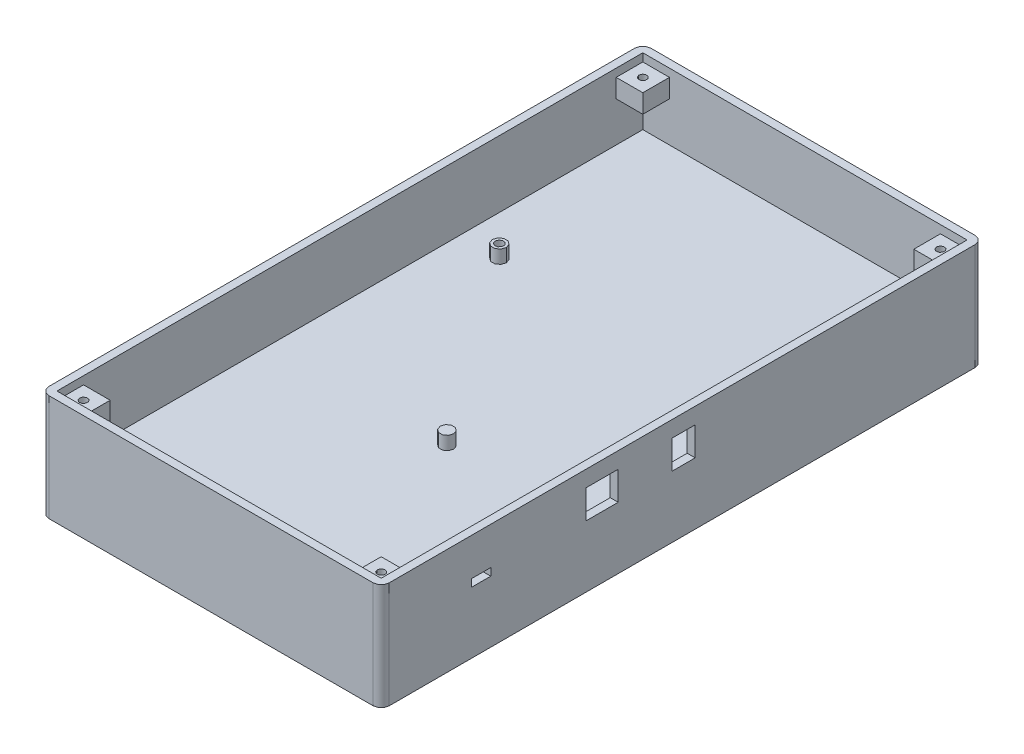
# Autodesk Inventor part: Base
Saved by Autodesk Inventor 2023 (Build 270158000, 158)
## iProperties
Created: 2023-01-13
Part Number: Base
Material: Generic
Document SubType Name: Modeling
Designer: Ahmed Nazir
Density: 1 g/cm^3
Appearance: Default
Author: Ahmed Nazir
Autodesk Inventor part; units mm, degrees
ref_plane "YZ Plane" through (0, 0, 0) normal (1, 0, 0) x (0, 1, 0)
ref_plane "XZ Plane" through (0, 0, 0) normal (0, 1, 0) x (-1, 0, 0)
ref_plane "XY Plane" through (0, 0, 0) normal (0, 0, 1) x (1, 0, 0)
sketch "Sketch1" plane through (0, 0, 0) normal (0, 1, 0) x (-1, 0, 0)
  line L0 (0, 0) -> (121.76, 0)
  line L1 (121.76, 0) -> (121.76, -220)
  line L2 (121.76, -220) -> (0, -220)
  line L3 (0, -220) -> (0, 0)
  line L4 (124.76, -223) -> (124.76, 3)
  line L5 (124.76, 3) -> (-3, 3)
  line L6 (-3, 3) -> (-3, -223)
  line L7 (-3, -223) -> (124.76, -223)
  circle A0 centre (5.08, -10.08) radius 1.6
  circle A1 centre (5.08, -10.08) radius 2.6
  circle A2 centre (55.88, -80.565) radius 2.5
  circle A3 centre (5.08, -151.05) radius 1.6
  circle A4 centre (5.08, -151.05) radius 2.6
  circle A5 centre (106.68, -10.08) radius 1.6
  circle A6 centre (106.68, -10.08) radius 2.6
  circle A7 centre (106.68, -151.05) radius 1.6
  circle A8 centre (106.68, -151.05) radius 2.6
  dimension "d0" = 121.76
  dimension "d1" = 220
  dimension "d2" = 3
  dimension "d22" = 3.2
  dimension "d23" = 1
  dimension "d24" = 5.08
  dimension "d25" = 10.08
  dimension "d26" = 5
  dimension "d35" = 3.2
  dimension "d36" = 1
  dimension "d37" = 140.97
  dimension "d38" = 0
  dimension "d39" = 3.2
  dimension "d40" = 1
  dimension "d41" = 101.6
  dimension "d42" = 0
  dimension "d43" = 3.2
  dimension "d44" = 1
  dimension "d45" = 0
  dimension "d46" = 0
  dimension "d47" = 50.8
  dimension "d48" = 70.485
  constraints: 16 end point, 9 centre point, 4 parallel, 2 perpendicular, 1 horizontal, 3 other
  measures "d0" distance of L1.end L2.end
  measures "d1" distance of L0.end L1.end
  measures "d2" distance between parallel lines of L1 L4
  measures "d22" diameter of A0
  measures "d23" radial gap between concentric circles of A0 A1
  measures "d24" distance from line of L3 A0.centre
  measures "d25" distance from line of A0.centre L0
  measures "d26" diameter of A2
  measures "d35" diameter of A3
  measures "d36" radial gap between concentric circles of A3 A4
  measures "d37" distance of A3.centre A0.centre
  measures "d38" horizontal distance of A3.centre A0.centre
  measures "d39" diameter of A5
  measures "d40" radial gap between concentric circles of A5 A6
  measures "d41" distance of A0.centre A5.centre
  measures "d42" vertical distance of A5.centre A0.centre
  measures "d43" diameter of A7
  measures "d44" radial gap between concentric circles of A7 A8
  measures "d45" vertical distance of A3.centre A7.centre
  measures "d46" horizontal distance of A5.centre A7.centre
  measures "d47" horizontal distance of A2.centre A0.centre
  measures "d48" vertical distance of A2.centre A5.centre
extrude "Extrusion1" add sketch "Sketch1" along normal blind 15 contours L0 L1 L2 L3 | A0 | A1 | A2 | A3 | A4 | A5 | A6 | A7 | A8
extrude "Extrusion2" add sketch "Sketch1" along normal blind 40 contours L7 L6 L5 L4
fillet "Fillet1" radius 3 4 edges at (3, 20, -223) (-124.76, 20, -223) (-124.76, 20, 3) (3, 20, 3)
sketch "Sketch2" plane through (3, 0, 0) normal (1, 0, 0) x (0, 0, -1)
  line L0 (220, 15) -> (0, 15) construction
  line L1 (0, 15) -> (220, 15)
  line L2 (73.9, 33.95) -> (86, 33.95)
  line L3 (86, 33.95) -> (86, 23.2)
  line L4 (86, 23.2) -> (73.9, 23.2)
  line L5 (73.9, 23.2) -> (73.9, 33.95)
  line L6 (106.15, 33.95) -> (114.9, 33.95)
  line L7 (114.9, 33.95) -> (114.9, 23.2)
  line L8 (114.9, 23.2) -> (106.15, 23.2)
  line L9 (106.15, 23.2) -> (106.15, 33.95)
  line L10 (0, 0) -> (0, 40) projected
  line L11 (30.85, 25.9) -> (38.15, 25.9)
  line L12 (38.15, 25.9) -> (38.15, 23.1)
  line L13 (38.15, 23.1) -> (30.85, 23.1)
  line L14 (30.85, 23.1) -> (30.85, 25.9)
  line L15 (110, 15) -> (110, 0) construction
  line L16 (220, 0) -> (0, 0) projected
  line L17 (48.413, 0) -> (43.7499, 10)
  line L18 (43.7499, 10) -> (66.2501, 10)
  line L19 (66.2501, 10) -> (61.587, 0)
  line L20 (48.413, 0) -> (61.587, 0)
  line L21 (55, 0) -> (55, 15) construction
  line L22 (171.587, 0) -> (176.2501, 10)
  line L23 (176.2501, 10) -> (153.7499, 10)
  line L24 (153.7499, 10) -> (158.413, 0)
  line L25 (171.587, 0) -> (158.413, 0)
  point P0 (110, 7.5)
  point P1 (55, 0)
  point P2 (158.413, 0)
  dimension "d9" = 12.1
  dimension "d10" = 10.75
  dimension "d11" = 8.2
  dimension "d12" = 8.75
  dimension "d13" = 10.75
  dimension "d14" = 8.2
  dimension "d15" = 20.15
  dimension "d19" = 7.3
  dimension "d20" = 2.8
  dimension "d21" = 8.1
  dimension "d49" = 35.75
  dimension "d50" = 30.85
  dimension "d72" = 13.174
  dimension "d73" = 65
  dimension "d74" = 65
  dimension "d75" = 10
  dimension "d76" = 55
  constraints: 46 end point, 7 equal length, 5 horizontal, 5 point on line, 4 midpoint, 4 perpendicular, 4 symmetric about line
  measures "d9" distance of L3.end L4.end
  measures "d10" distance of L2.end L3.end
  measures "d11" distance between parallel lines of L0 L4
  measures "d12" distance of L7.end L8.end
  measures "d13" distance of L6.end L7.end
  measures "d14" distance between parallel lines of L0 L8
  measures "d15" distance between parallel lines of L9 L3
  measures "d19" distance of L12.end L13.end
  measures "d20" distance of L11.end L12.end
  measures "d21" distance between parallel lines of L0 L13
  measures "d49" distance between parallel lines of L5 L12
  measures "d50" distance between parallel lines of L10 L14
  measures "d72" distance of L17.start L19.end
  measures "d73" angle of L16 L19
  measures "d74" angle of L16 L17
  measures "d75" distance between parallel lines of L20 L18
  measures "d76" distance from line of point (110, 7.5) L21
extrude "Extrusion3" cut sketch "Sketch2" against normal up to surface (3 mm away) contours L2 L3 L4 L5 | L6 L7 L8 L9 | L11 L12 L13 L14
extrude "Extrusion4" add sketch "Sketch1" along normal blind 20 contours A1 | A2 | A4 | A6 | A8
sketch "Sketch3" plane through (0, 40, 0) normal (0, 1, 0) x (1, 0, 0)
  line L0 (-121.76, 0) -> (-121.76, 220) projected
  line L1 (-121.76, 110) -> (0, 110) construction
  line L2 (0, 220) -> (0, 0) projected
  line L3 (-121.76, 0) -> (0, 0) projected
  line L4 (-60.88, 0) -> (-60.88, 220) construction
  line L5 (-121.76, 220) -> (0, 220) projected
  line L6 (0, 0) -> (-10, 0)
  line L7 (-10, 0) -> (-10, 10)
  line L8 (-10, 10) -> (0, 10)
  line L9 (0, 10) -> (0, 0)
  line L10 (-121.76, 0) -> (-111.76, 0)
  line L11 (-111.76, 0) -> (-111.76, 10)
  line L12 (-111.76, 10) -> (-121.76, 10)
  line L13 (-121.76, 10) -> (-121.76, 0)
  line L14 (0, 220) -> (-10, 220)
  line L15 (-10, 220) -> (-10, 210)
  line L16 (-10, 210) -> (0, 210)
  line L17 (0, 210) -> (0, 220)
  line L18 (-121.76, 220) -> (-111.76, 220)
  line L19 (-111.76, 220) -> (-111.76, 210)
  line L20 (-111.76, 210) -> (-121.76, 210)
  line L21 (-121.76, 210) -> (-121.76, 220)
  line L22 (-121.76, 0) -> (0, 0)
  line L23 (0, 0) -> (0, 220)
  line L24 (0, 220) -> (-121.76, 220)
  line L25 (-121.76, 220) -> (-121.76, 0)
  point P0 (0, 210)
  dimension "d51" = 10
  dimension "d52" = 10
  constraints: 44 end point, 9 symmetric about line, 4 midpoint, 4 parallel, 2 horizontal, 2 perpendicular
  measures "d51" distance of L7.end L8.end
  measures "d52" distance of L6.end L7.end
extrude "Extrusion6" add sketch "Sketch3" against normal blind 10 contours L0 L12 L11 L3 | L0 L5 L19 L20 | L7 L8 L2 L3 | L5 L2 L16 L15
sketch "Sketch4" plane through (0, 40, 0) normal (0, 1, 0) x (1, 0, 0)
  line L0 (-10, 10) -> (-10, 0) projected
  line L1 (0, 10) -> (-10, 10) projected
  line L2 (-10, 220) -> (-10, 210) projected
  line L3 (-10, 210) -> (0, 210) projected
  line L4 (-121.76, 210) -> (-111.76, 210) projected
  line L5 (-111.76, 210) -> (-111.76, 220) projected
  line L6 (-111.76, 0) -> (-111.76, 10) projected
  line L7 (-111.76, 10) -> (-121.76, 10) projected
  point P0 (0, 0)
  point P1 (-5, 5)
  point P2 (-116.76, 5)
  point P3 (-116.76, 215)
  point P4 (-5, 215)
  dimension "d55" = 5
  dimension "d63" = 5
  dimension "d64" = 5
  dimension "d65" = 5
  dimension "d66" = 5
  dimension "d67" = 5
  dimension "d68" = 5
  dimension "d69" = 5
  measures "d55" distance from line of L0 point (-5, 5)
  measures "d63" distance from line of L1 point (-5, 5)
  measures "d64" distance from line of L2 point (-5, 215)
  measures "d65" distance from line of L3 point (-5, 215)
  measures "d66" distance from line of L4 point (-116.76, 215)
  measures "d67" distance from line of L5 point (-116.76, 215)
  measures "d68" distance from line of L6 point (-116.76, 5)
  measures "d69" distance from line of L7 point (-116.76, 5)
hole "Hole1" at (-5, 40, -5) at (-5, 40, -215) at (-116.76, 40, -215) at (-116.76, 40, -5) direction (0, -1, 0) diameter 3 depth 10
extrude "Extrusion7" cut sketch "Sketch3" against normal blind 3
extrude "Extrusion8" cut sketch "Sketch2" against normal up to surface (127.76 mm away) contours L16 L17 L18 L19 | L16 L24 L23 L22
extrude "Extrusion9" add sketch "Sketch2" against normal blind 2.5 contours L16 L17 L18 L19 | L16 L24 L23 L22
sketch "Sketch5" plane through (-121.76, 0, 3) normal (0, 0, 1) x (1, 0, 0)
  line L0 (122.26, 10) -> (-3, 10) projected
  line L1 (59.63, 10) -> (59.63, 0) construction
  line L2 (-3, 0) -> (122.26, 0) projected
  line L3 (29.815, 10) -> (29.815, 0) construction
  line L4 (23.228, 0) -> (36.402, 0)
  line L5 (36.402, 0) -> (41.0651, 10)
  line L6 (41.0651, 10) -> (18.5649, 10)
  line L7 (18.5649, 10) -> (23.228, 0)
  line L8 (89.445, 10) -> (89.445, 0) construction
  line L9 (96.032, 0) -> (82.858, 0)
  line L10 (82.858, 0) -> (78.1949, 10)
  line L11 (78.1949, 10) -> (100.6951, 10)
  line L12 (100.6951, 10) -> (96.032, 0)
  point P0 (121.76, 0)
  point P1 (59.63, 5)
  point P2 (18.5649, 10)
  point P3 (41.0651, 10)
  dimension "d81" = 29.815
  dimension "d82" = 13.174
  dimension "d83" = 65
  dimension "d84" = 65
  dimension "d85" = 10
  constraints: 22 end point, 7 symmetric about line, 6 point on line, 4 midpoint, 1 parallel, 1 perpendicular
  measures "d81" distance from line of point (59.63, 5) L3
  measures "d82" distance of L4.start L4.end
  measures "d83" angle of L2 L5
  measures "d84" angle of L2 L7
  measures "d85" distance between parallel lines of L2 L6
extrude "Extrusion10" cut sketch "Sketch5" against normal up to surface (226 mm away) contours L12 L2 L10 L0 | L5 L2 L7 L0
extrude "Extrusion11" add sketch "Sketch5" against normal blind 2.5 contours L12 L2 L10 L0 | L5 L2 L7 L0
body "Solid1"
